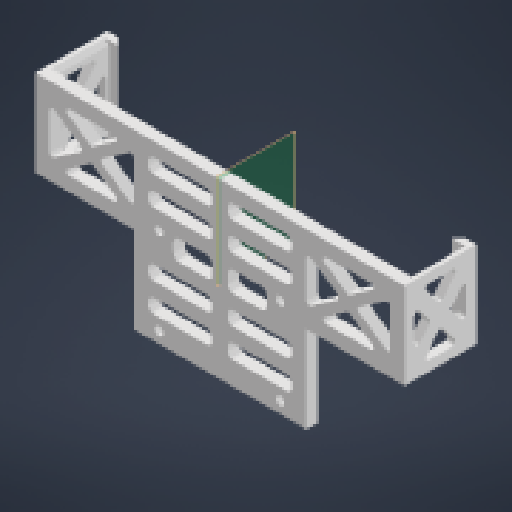
# Autodesk Inventor part: Mux_switch_holder
Saved by Autodesk Inventor 2026.1 (Build 301233020, 233B)
## iProperties
Created: 2025-10-27
Part Number: Mux_switch_holder
Material: Generic
Document SubType Name: Modeling
Designer: Mikke
Density: 1 g/cm^3
Appearance: Default
Author: Mikke
Autodesk Inventor part; units mm, degrees
(part 1 of 2)
ref_plane "YZ Plane" through (0, 0, 0) normal (1, 0, 0) x (0, 1, 0)
ref_plane "XZ Plane" through (0, 0, 0) normal (0, 1, 0) x (-1, 0, 0)
ref_plane "XY Plane" through (0, 0, 0) normal (0, 0, 1) x (1, 0, 0)
sketch "Sketch1" plane through (0, 0, 0) normal (0, 0, 1) x (1, 0, 0)
  line L0 (44.8879, -29.1603) -> (44.2305, -29.1603) projected
  line L1 (44.2305, -29.1603) -> (44.2305, -28.4336) projected
  line L2 (44.2305, -28.4336) -> (42.1345, -28.4336) projected
  line L3 (42.1345, -28.4336) -> (42.1345, -27.6476) projected
  line L4 (42.1345, -27.6476) -> (44.2305, -27.6476) projected
  line L5 (44.2305, -27.6476) -> (44.2305, -24.9536) projected
  line L6 (44.2305, -24.9536) -> (45.0906, -24.9536) projected
  line L7 (45.0906, -24.9536) -> (48.2345, -27.6822) projected
  line L8 (48.2345, -27.6822) -> (48.2345, -28.4336) projected
  line L9 (48.2345, -28.4336) -> (44.8879, -28.4336) projected
  line L10 (44.8879, -28.4336) -> (44.8879, -29.1603) projected
  line L11 (44.4529, -11.8242) -> (42.1345, -13.4011) projected
  line L12 (42.1345, -13.4011) -> (42.1345, -12.457) projected
  line L13 (42.1345, -12.457) -> (43.8548, -11.3447) projected
  line L14 (43.8548, -11.3447) -> (42.1345, -10.2028) projected
  line L15 (42.1345, -10.2028) -> (42.1345, -9.3279) projected
  line L16 (42.1345, -9.3279) -> (44.4035, -10.9147) projected
  line L17 (44.4035, -10.9147) -> (46.712, -9.3427) projected
  line L18 (46.712, -9.3427) -> (46.712, -10.2869) projected
  line L19 (46.712, -10.2869) -> (45.0065, -11.3942) projected
  line L20 (45.0065, -11.3942) -> (46.712, -12.5262) projected
  line L21 (46.712, -12.5262) -> (46.712, -13.4011) projected
  line L22 (46.712, -13.4011) -> (44.4529, -11.8242) projected
  line L23 (46.712, -8.7149) -> (42.1345, -8.7149) projected
  line L24 (42.1345, -8.7149) -> (42.1345, -7.9438) projected
  line L25 (42.1345, -7.9438) -> (46.712, -7.9438) projected
  line L26 (46.712, -7.9438) -> (46.712, -8.7149) projected
  spline S0 degree 2 poles (42.1741, -4.3352) (42.1147, -4.1177) (42.0455, -3.6728) (42.0455, -3.48) knots 0 0 0 1 2 2 2 projected
  spline S1 degree 2 poles (42.0455, -3.48) (42.0455, -2.8522) (42.7623, -2.1453) (43.5384, -2.1453) knots 0 0 0 1 2 2 2 projected
  line L27 (43.5384, -2.1453) -> (46.0743, -2.1453) projected
  line L28 (46.0743, -2.1453) -> (46.0743, -1.6262) projected
  line L29 (46.0743, -1.6262) -> (46.712, -1.6262) projected
  line L30 (46.712, -1.6262) -> (46.712, -2.1453) projected
  line L31 (46.712, -2.1453) -> (48.0269, -2.1453) projected
  line L32 (48.0269, -2.1453) -> (48.0269, -2.9164) projected
  line L33 (48.0269, -2.9164) -> (46.712, -2.9164) projected
  line L34 (46.712, -2.9164) -> (46.712, -4.3352) projected
  line L35 (46.712, -4.3352) -> (46.0743, -4.3352) projected
  line L36 (46.0743, -4.3352) -> (46.0743, -2.9164) projected
  line L37 (46.0743, -2.9164) -> (43.8943, -2.9164) projected
  spline S2 degree 2 poles (43.8943, -2.9164) (43.5483, -2.9164) (43.1676, -2.9412) (43.0045, -3.0252) knots 0 0 0 1 2 2 2 projected
  spline S3 degree 2 poles (43.0045, -3.0252) (42.8612, -3.0944) (42.7178, -3.4058) (42.7178, -3.6728) knots 0 0 0 1 2 2 2 projected
  spline S4 degree 2 poles (42.7178, -3.6728) (42.7178, -3.8606) (42.8315, -4.2116) (42.8661, -4.2907) knots 0 0 0 1 2 2 2 projected
  line L38 (42.8661, -4.2907) -> (42.8661, -4.3352) projected
  line L39 (42.8661, -4.3352) -> (42.1741, -4.3352) projected
  line L40 (42.1345, -0.2421) -> (42.6189, -0.2421) projected
  spline S5 degree 2 poles (42.6189, -0.2421) (42.5497, -0.1482) (42.3026, 0.1682) (42.2284, 0.3165) knots 0 0 0 1 2 2 2 projected
  spline S6 degree 2 poles (42.2284, 0.3165) (42.1197, 0.5191) (42.006, 0.8998) (42.006, 1.2458) knots 0 0 0 1 2 2 2 projected
  spline S7 degree 2 poles (42.006, 1.2458) (42.006, 1.5276) (42.2185, 2.0367) (42.4113, 2.2295) knots 0 0 0 1 2 2 2 projected
  spline S8 degree 2 poles (42.4113, 2.2295) (42.5992, 2.4124) (43.1528, 2.6349) (43.4593, 2.6349) knots 0 0 0 1 2 2 2 projected
  spline S9 degree 2 poles (43.4593, 2.6349) (43.9339, 2.6349) (44.6061, 2.2344) (44.7989, 1.7994) knots 0 0 0 1 2 2 2 projected
  spline S10 degree 2 poles (44.7989, 1.7994) (44.9769, 1.4139) (45.1104, 0.3659) (45.145, -0.2421) knots 0 0 0 1 2 2 2 projected
  line L41 (45.145, -0.2421) -> (45.2933, -0.2421) projected
  spline S11 degree 2 poles (45.2933, -0.2421) (45.5602, -0.2421) (45.8914, -0.079) (45.9853, 0.0693) knots 0 0 0 1 2 2 2 projected
  spline S12 degree 2 poles (45.9853, 0.0693) (46.0792, 0.2176) (46.1386, 0.6427) (46.1386, 0.8701) knots 0 0 0 1 2 2 2 projected
  spline S13 degree 2 poles (46.1386, 0.8701) (46.1386, 1.137) (45.9804, 1.8588) (45.8271, 2.2196) knots 0 0 0 1 2 2 2 projected
  line L42 (45.8271, 2.2196) -> (45.8271, 2.2641) projected
  line L43 (45.8271, 2.2641) -> (46.6131, 2.2641) projected
  spline S14 degree 2 poles (46.6131, 2.2641) (46.6724, 2.0515) (46.8207, 1.2557) (46.8207, 0.8652) knots 0 0 0 1 2 2 2 projected
  spline S15 degree 2 poles (46.8207, 0.8652) (46.8207, 0.3906) (46.6724, -0.257) (46.4796, -0.514) knots 0 0 0 1 2 2 2 projected
  spline S16 degree 2 poles (46.4796, -0.514) (46.2918, -0.7661) (45.6937, -1.0133) (45.2636, -1.0133) knots 0 0 0 1 2 2 2 projected
  line L44 (45.2636, -1.0133) -> (42.1345, -1.0133) projected
  line L45 (42.1345, -1.0133) -> (42.1345, -0.2421) projected
  line L46 (46.6873, 11.9925) -> (45.8865, 11.9925) projected
  line L47 (45.8865, 11.9925) -> (45.8865, 12.032) projected
  spline S17 degree 2 poles (45.8865, 12.032) (45.9112, 12.121) (45.9211, 12.3138) (45.9211, 12.4473) knots 0 0 0 1 2 2 2 projected
  spline S18 degree 2 poles (45.9211, 12.4473) (45.9211, 12.7587) (45.6492, 13.3716) (45.3822, 13.6485) knots 0 0 0 1 2 2 2 projected
  line L48 (45.3822, 13.6485) -> (42.1345, 13.6485) projected
  line L49 (42.1345, 13.6485) -> (42.1345, 14.4196) projected
  line L50 (42.1345, 14.4196) -> (46.712, 14.4196) projected
  line L51 (46.712, 14.4196) -> (46.712, 13.6485) projected
  line L52 (46.712, 13.6485) -> (46.0298, 13.6485) projected
  spline S19 degree 2 poles (46.0298, 13.6485) (46.4055, 13.2283) (46.712, 12.6005) (46.712, 12.3039) knots 0 0 0 1 2 2 2 projected
  spline S20 degree 2 poles (46.712, 12.3039) (46.712, 12.1853) (46.7021, 12.0666) (46.6873, 11.9925) knots 0 0 0 1 2 2 2 projected
  spline S21 degree 2 poles (42.1592, 15.9817) (42.095, 16.2041) (42.0307, 16.5699) (42.0307, 16.8468) knots 0 0 0 1 2 2 2 projected
  spline S22 degree 2 poles (42.0307, 16.8468) (42.0307, 17.9442) (43.2616, 19.1503) (44.3985, 19.1503) knots 0 0 0 1 2 2 2 projected
  spline S23 degree 2 poles (44.3985, 19.1503) (45.5157, 19.1503) (46.8405, 17.9788) (46.8405, 17.0346) knots 0 0 0 1 2 2 2 projected
  spline S24 degree 2 poles (46.8405, 17.0346) (46.8405, 16.6095) (46.5933, 15.952) (46.3313, 15.7098) knots 0 0 0 1 2 2 2 projected
  spline S25 degree 2 poles (46.3313, 15.7098) (46.0694, 15.4626) (45.313, 15.2007) (44.7643, 15.2007) knots 0 0 0 1 2 2 2 projected
  line L53 (44.7643, 15.2007) -> (44.3441, 15.2007) projected
  line L54 (44.3441, 15.2007) -> (44.3441, 18.3693) projected
  spline S26 degree 2 poles (44.3441, 18.3693) (43.5483, 18.3693) (42.703, 17.5685) (42.703, 16.8567) knots 0 0 0 1 2 2 2 projected
  spline S27 degree 2 poles (42.703, 16.8567) (42.703, 16.6045) (42.8167, 16.1152) (42.9057, 15.9174) knots 0 0 0 1 2 2 2 projected
  spline S28 degree 2 poles (42.9057, 15.9174) (43.0045, 15.7098) (43.1775, 15.4231) (43.2566, 15.3292) knots 0 0 0 1 2 2 2 projected
  line L55 (43.2566, 15.3292) -> (43.2566, 15.2847) projected
  line L56 (43.2566, 15.2847) -> (42.4163, 15.2847) projected
  spline S29 degree 2 poles (42.4163, 15.2847) (42.3619, 15.4182) (42.2037, 15.8235) (42.1592, 15.9817) knots 0 0 0 1 2 2 2 projected
  spline S30 degree 2 poles (42.1741, 21.3204) (42.1147, 21.5379) (42.0455, 21.9828) (42.0455, 22.1756) knots 0 0 0 1 2 2 2 projected
  spline S31 degree 2 poles (42.0455, 22.1756) (42.0455, 22.8034) (42.7623, 23.5103) (43.5384, 23.5103) knots 0 0 0 1 2 2 2 projected
  line L57 (43.5384, 23.5103) -> (46.0743, 23.5103) projected
  line L58 (46.0743, 23.5103) -> (46.0743, 24.0293) projected
  line L59 (46.0743, 24.0293) -> (46.712, 24.0293) projected
  line L60 (46.712, 24.0293) -> (46.712, 23.5103) projected
  line L61 (46.712, 23.5103) -> (48.0269, 23.5103) projected
  line L62 (48.0269, 23.5103) -> (48.0269, 22.7391) projected
  line L63 (48.0269, 22.7391) -> (46.712, 22.7391) projected
  line L64 (46.712, 22.7391) -> (46.712, 21.3204) projected
  line L65 (46.712, 21.3204) -> (46.0743, 21.3204) projected
  line L66 (46.0743, 21.3204) -> (46.0743, 22.7391) projected
  line L67 (46.0743, 22.7391) -> (43.8943, 22.7391) projected
  spline S32 degree 2 poles (43.8943, 22.7391) (43.5483, 22.7391) (43.1676, 22.7144) (43.0045, 22.6304) knots 0 0 0 1 2 2 2 projected
  spline S33 degree 2 poles (43.0045, 22.6304) (42.8612, 22.5612) (42.7178, 22.2498) (42.7178, 21.9828) knots 0 0 0 1 2 2 2 projected
  spline S34 degree 2 poles (42.7178, 21.9828) (42.7178, 21.795) (42.8315, 21.444) (42.8661, 21.3649) knots 0 0 0 1 2 2 2 projected
  line L68 (42.8661, 21.3649) -> (42.8661, 21.3204) projected
  line L69 (42.8661, 21.3204) -> (42.1741, 21.3204) projected
  spline S35 degree 2 poles (45.5256, 30.1244) (45.3773, 29.5806) (44.5913, 28.9825) (44.008, 28.9825) knots 0 0 0 1 2 2 2 projected
  spline S36 degree 2 poles (44.008, 28.9825) (43.5532, 28.9825) (42.8562, 29.3285) (42.6288, 29.6152) knots 0 0 0 1 2 2 2 projected
  spline S37 degree 2 poles (42.6288, 29.6152) (42.3619, 29.9613) (42.1345, 30.7473) (42.1345, 31.3701) knots 0 0 0 1 2 2 2 projected
  line L70 (42.1345, 31.3701) -> (42.1345, 33.12) projected
  line L71 (42.1345, 33.12) -> (48.2345, 33.12) projected
  line L72 (48.2345, 33.12) -> (48.2345, 31.5036) projected
  spline S38 degree 2 poles (48.2345, 31.5036) (48.2345, 30.8511) (48.1505, 30.1985) (47.9873, 29.902) knots 0 0 0 1 2 2 2 projected
  spline S39 degree 2 poles (47.9873, 29.902) (47.8143, 29.5708) (47.2459, 29.2692) (46.8603, 29.2692) knots 0 0 0 1 2 2 2 projected
  spline S40 degree 2 poles (46.8603, 29.2692) (46.4302, 29.2692) (45.748, 29.724) (45.5553, 30.1244) knots 0 0 0 1 2 2 2 projected
  line L73 (45.5553, 30.1244) -> (45.5256, 30.1244) projected
  line L74 (52.8849, -32.3388) -> (52.178, -32.3388) projected
  line L75 (52.178, -32.3388) -> (52.178, -28.577) projected
  line L76 (52.178, -28.577) -> (53.0431, -28.577) projected
  spline S41 degree 2 poles (53.0431, -28.577) (53.4237, -28.9823) (54.1306, -29.704) (54.5112, -30.0501) knots 0 0 0 1 2 2 2 projected
  spline S42 degree 2 poles (54.5112, -30.0501) (55.2774, -30.7471) (56.1969, -31.2562) (56.6863, -31.2562) knots 0 0 0 1 2 2 2 projected
  spline S43 degree 2 poles (56.6863, -31.2562) (56.9433, -31.2562) (57.3289, -31.098) (57.4525, -30.9547) knots 0 0 0 1 2 2 2 projected
  spline S44 degree 2 poles (57.4525, -30.9547) (57.5761, -30.8113) (57.6996, -30.4357) (57.6996, -30.2083) knots 0 0 0 1 2 2 2 projected
  spline S45 degree 2 poles (57.6996, -30.2083) (57.6996, -29.9908) (57.5909, -29.5459) (57.5068, -29.3432) knots 0 0 0 1 2 2 2 projected
  spline S46 degree 2 poles (57.5068, -29.3432) (57.4376, -29.1702) (57.2399, -28.8489) (57.1707, -28.75) knots 0 0 0 1 2 2 2 projected
  line L77 (57.1707, -28.75) -> (57.1707, -28.7055) projected
  line L78 (57.1707, -28.7055) -> (58.0407, -28.7055) projected
  spline S47 degree 2 poles (58.0407, -28.7055) (58.1643, -28.9576) (58.4065, -29.8622) (58.4065, -30.2676) knots 0 0 0 1 2 2 2 projected
  spline S48 degree 2 poles (58.4065, -30.2676) (58.4065, -31.1228) (57.5019, -32.0867) (56.7308, -32.0867) knots 0 0 0 1 2 2 2 projected
  spline S49 degree 2 poles (56.7308, -32.0867) (56.3699, -32.0867) (55.7668, -31.9186) (55.5098, -31.7703) knots 0 0 0 1 2 2 2 projected
  spline S50 degree 2 poles (55.5098, -31.7703) (55.2428, -31.622) (54.7188, -31.192) (54.4667, -30.9547) knots 0 0 0 1 2 2 2 projected
  spline S51 degree 2 poles (54.4667, -30.9547) (54.0466, -30.5691) (53.1469, -29.625) (52.8849, -29.3432) knots 0 0 0 1 2 2 2 projected
  line L79 (52.8849, -29.3432) -> (52.8849, -32.3388) projected
  line L80 (55.2181, -23.1888) -> (54.4766, -23.1888) projected
  line L81 (54.4766, -23.1888) -> (54.4766, -20.8803) projected
  line L82 (54.4766, -20.8803) -> (55.2181, -20.8803) projected
  line L83 (55.2181, -20.8803) -> (55.2181, -23.1888) projected
  line L84 (55.2181, -15.5663) -> (54.4766, -15.5663) projected
  line L85 (54.4766, -15.5663) -> (54.4766, -13.2578) projected
  line L86 (54.4766, -13.2578) -> (55.2181, -13.2578) projected
  line L87 (55.2181, -13.2578) -> (55.2181, -15.5663) projected
  line L88 (52.178, -7.9438) -> (52.178, -4.1275) projected
  line L89 (52.178, -4.1275) -> (58.278, -4.1275) projected
  line L90 (58.278, -4.1275) -> (58.278, -7.9438) projected
  line L91 (58.278, -7.9438) -> (57.5563, -7.9438) projected
  line L92 (57.5563, -7.9438) -> (57.5563, -4.9382) projected
  line L93 (57.5563, -4.9382) -> (55.8855, -4.9382) projected
  line L94 (55.8855, -4.9382) -> (55.8855, -7.7411) projected
  line L95 (55.8855, -7.7411) -> (55.1637, -7.7411) projected
  line L96 (55.1637, -7.7411) -> (55.1637, -4.9382) projected
  line L97 (55.1637, -4.9382) -> (52.8997, -4.9382) projected
  line L98 (52.8997, -4.9382) -> (52.8997, -7.9438) projected
  line L99 (52.8997, -7.9438) -> (52.178, -7.9438) projected
  line L100 (52.8008, 10.1931) -> (52.178, 10.1931) projected
  line L101 (52.178, 10.1931) -> (52.178, 13.169) projected
  line L102 (52.178, 13.169) -> (52.8008, 13.169) projected
  line L103 (52.8008, 13.169) -> (52.8008, 12.0617) projected
  line L104 (52.8008, 12.0617) -> (56.8889, 12.0617) projected
  line L105 (56.8889, 12.0617) -> (56.8889, 13.169) projected
  line L106 (56.8889, 13.169) -> (57.4475, 13.169) projected
  spline S52 degree 2 poles (57.4475, 13.169) (57.4475, 12.5412) (57.8034, 11.948) (58.2978, 11.9084) knots 0 0 0 1 2 2 2 projected
  line L107 (58.2978, 11.9084) -> (58.2978, 11.2757) projected
  line L108 (58.2978, 11.2757) -> (52.8008, 11.2757) projected
  line L109 (52.8008, 11.2757) -> (52.8008, 10.1931) projected
  spline S53 degree 2 poles (52.6229, 25.1218) (52.356, 25.4135) (52.0692, 26.155) (52.0692, 26.7135) knots 0 0 0 1 2 2 2 projected
  spline S54 degree 2 poles (52.0692, 26.7135) (52.0692, 27.3759) (52.3461, 28.3053) (52.5438, 28.7156) knots 0 0 0 1 2 2 2 projected
  line L110 (52.5438, 28.7156) -> (53.5621, 28.7156) projected
  line L111 (53.5621, 28.7156) -> (53.5621, 28.6562) projected
  spline S55 degree 2 poles (53.5621, 28.6562) (53.1864, 28.2558) (52.7712, 27.2425) (52.7712, 26.7729) knots 0 0 0 1 2 2 2 projected
  spline S56 degree 2 poles (52.7712, 26.7729) (52.7712, 26.1006) (53.3298, 25.4135) (53.7895, 25.4135) knots 0 0 0 1 2 2 2 projected
  spline S57 degree 2 poles (53.7895, 25.4135) (54.1553, 25.4135) (54.6101, 25.7743) (54.7238, 26.1648) knots 0 0 0 1 2 2 2 projected
  spline S58 degree 2 poles (54.7238, 26.1648) (54.8029, 26.4466) (54.9116, 26.9162) (55.0006, 27.2672) knots 0 0 0 1 2 2 2 projected
  spline S59 degree 2 poles (55.0006, 27.2672) (55.0846, 27.5836) (55.3367, 28.0828) (55.5394, 28.2756) knots 0 0 0 1 2 2 2 projected
  spline S60 degree 2 poles (55.5394, 28.2756) (55.7421, 28.4635) (56.2859, 28.6711) (56.6418, 28.6711) knots 0 0 0 1 2 2 2 projected
  spline S61 degree 2 poles (56.6418, 28.6711) (57.3833, 28.6711) (58.3867, 27.5144) (58.3867, 26.6196) knots 0 0 0 1 2 2 2 projected
  spline S62 degree 2 poles (58.3867, 26.6196) (58.3867, 26.1055) (58.1841, 25.196) (57.9913, 24.8054) knots 0 0 0 1 2 2 2 projected
  line L112 (57.9913, 24.8054) -> (57.0224, 24.8054) projected
  line L113 (57.0224, 24.8054) -> (57.0224, 24.8648) projected
  spline S63 degree 2 poles (57.0224, 24.8648) (57.2893, 25.1564) (57.6848, 26.066) (57.6848, 26.5652) knots 0 0 0 1 2 2 2 projected
  spline S64 degree 2 poles (57.6848, 26.5652) (57.6848, 27.1288) (57.1559, 27.8258) (56.7258, 27.8258) knots 0 0 0 1 2 2 2 projected
  spline S65 degree 2 poles (56.7258, 27.8258) (56.3402, 27.8258) (55.8805, 27.4155) (55.7767, 27.0299) knots 0 0 0 1 2 2 2 projected
  spline S66 degree 2 poles (55.7767, 27.0299) (55.7075, 26.7729) (55.5295, 26.0264) (55.4554, 25.7793) knots 0 0 0 1 2 2 2 projected
  spline S67 degree 2 poles (55.4554, 25.7793) (55.2626, 25.1515) (54.4865, 24.5682) (53.918, 24.5682) knots 0 0 0 1 2 2 2 projected
  spline S68 degree 2 poles (53.918, 24.5682) (53.5572, 24.5682) (52.8651, 24.8598) (52.6229, 25.1218) knots 0 0 0 1 2 2 2 projected
  line L114 (52.178, 29.3038) -> (52.178, 33.12) projected
  line L115 (52.178, 33.12) -> (58.278, 33.12) projected
  line L116 (58.278, 33.12) -> (58.278, 29.3038) projected
  line L117 (58.278, 29.3038) -> (57.5563, 29.3038) projected
  line L118 (57.5563, 29.3038) -> (57.5563, 32.3093) projected
  line L119 (57.5563, 32.3093) -> (55.8855, 32.3093) projected
  line L120 (55.8855, 32.3093) -> (55.8855, 29.5065) projected
  line L121 (55.8855, 29.5065) -> (55.1637, 29.5065) projected
  line L122 (55.1637, 29.5065) -> (55.1637, 32.3093) projected
  line L123 (55.1637, 32.3093) -> (52.8997, 32.3093) projected
  line L124 (52.8997, 32.3093) -> (52.8997, 29.3038) projected
  line L125 (52.8997, 29.3038) -> (52.178, 29.3038) projected
  spline S69 degree 2 poles (57.7936, 20.1686) (57.403, 19.5804) (56.1128, 18.9328) (55.2231, 18.9328) knots 0 0 0 1 2 2 2 projected
  spline S70 degree 2 poles (55.2231, 18.9328) (54.3876, 18.9328) (53.0431, 19.6101) (52.6674, 20.1785) knots 0 0 0 1 2 2 2 projected
  spline S71 degree 2 poles (52.6674, 20.1785) (52.3757, 20.6432) (52.178, 21.5973) (52.178, 22.3387) knots 0 0 0 1 2 2 2 projected
  line L126 (52.178, 22.3387) -> (52.178, 23.7426) projected
  line L127 (52.178, 23.7426) -> (58.278, 23.7426) projected
  line L128 (58.278, 23.7426) -> (58.278, 22.3536) projected
  spline S72 degree 2 poles (58.278, 22.3536) (58.278, 21.4934) (58.0209, 20.5147) (57.7936, 20.1686) knots 0 0 0 1 2 2 2 projected
  spline S73 degree 2 poles (55.5889, 15.1562) (55.3615, 14.8546) (54.6694, 14.5284) (54.1158, 14.5284) knots 0 0 0 1 2 2 2 projected
  spline S74 degree 2 poles (54.1158, 14.5284) (53.6758, 14.5284) (52.9244, 14.8101) (52.6476, 15.0672) knots 0 0 0 1 2 2 2 projected
  spline S75 degree 2 poles (52.6476, 15.0672) (52.3708, 15.3242) (52.0495, 16.0904) (52.0495, 16.565) knots 0 0 0 1 2 2 2 projected
  spline S76 degree 2 poles (52.0495, 16.565) (52.0495, 17) (52.2423, 17.8503) (52.3955, 18.1617) knots 0 0 0 1 2 2 2 projected
  line L129 (52.3955, 18.1617) -> (53.2606, 18.1617) projected
  line L130 (53.2606, 18.1617) -> (53.2606, 18.1024) projected
  spline S77 degree 2 poles (53.2606, 18.1024) (53.1914, 18.0084) (53.0134, 17.6575) (52.9343, 17.4449) knots 0 0 0 1 2 2 2 projected
  spline S78 degree 2 poles (52.9343, 17.4449) (52.8503, 17.2027) (52.7564, 16.8023) (52.7564, 16.5502) knots 0 0 0 1 2 2 2 projected
  spline S79 degree 2 poles (52.7564, 16.5502) (52.7564, 16.303) (52.9343, 15.8383) (53.1271, 15.6703) knots 0 0 0 1 2 2 2 projected
  spline S80 degree 2 poles (53.1271, 15.6703) (53.31, 15.517) (53.7944, 15.3588) (54.1207, 15.3588) knots 0 0 0 1 2 2 2 projected
  spline S81 degree 2 poles (54.1207, 15.3588) (54.447, 15.3588) (54.8622, 15.5368) (55.0006, 15.7049) knots 0 0 0 1 2 2 2 projected
  spline S82 degree 2 poles (55.0006, 15.7049) (55.1538, 15.8779) (55.2824, 16.392) (55.2824, 16.7034) knots 0 0 0 1 2 2 2 projected
  spline S83 degree 2 poles (55.2824, 16.7034) (55.2824, 17.0396) (55.1786, 17.7069) (55.1341, 17.9096) knots 0 0 0 1 2 2 2 projected
  line L131 (55.1341, 17.9096) -> (58.278, 17.9096) projected
  line L132 (58.278, 17.9096) -> (58.278, 14.563) projected
  line L133 (58.278, 14.563) -> (57.5612, 14.563) projected
  line L134 (57.5612, 14.563) -> (57.5612, 17.1236) projected
  line L135 (57.5612, 17.1236) -> (55.9349, 17.1236) projected
  spline S84 degree 2 poles (55.9349, 17.1236) (55.9547, 16.9753) (55.9695, 16.6886) (55.9695, 16.5699) knots 0 0 0 1 2 2 2 projected
  spline S85 degree 2 poles (55.9695, 16.5699) (55.9695, 16.1003) (55.8162, 15.4528) (55.5889, 15.1562) knots 0 0 0 1 2 2 2 projected
  spline S86 degree 2 poles (58.4016, 7.2222) (58.4016, 6.2187) (56.8197, 5.2746) (55.228, 5.2746) knots 0 0 0 1 2 2 2 projected
  spline S87 degree 2 poles (55.228, 5.2746) (53.5868, 5.2746) (52.0495, 6.2286) (52.0495, 7.2222) knots 0 0 0 1 2 2 2 projected
  spline S88 degree 2 poles (52.0495, 7.2222) (52.0495, 8.2306) (53.6165, 9.1748) (55.2231, 9.1748) knots 0 0 0 1 2 2 2 projected
  spline S89 degree 2 poles (55.2231, 9.1748) (56.8741, 9.1748) (58.4016, 8.2208) (58.4016, 7.2222) knots 0 0 0 1 2 2 2 projected
  line L136 (58.5499, 0.0396) -> (58.5499, -0.6623) projected
  line L137 (58.5499, -0.6623) -> (50.8532, 1.7253) projected
  line L138 (50.8532, 1.7253) -> (50.8532, 2.4173) projected
  line L139 (50.8532, 2.4173) -> (58.5499, 0.0396) projected
  spline S90 degree 2 poles (52.6229, -12.1258) (52.356, -11.8341) (52.0692, -11.0926) (52.0692, -10.534) knots 0 0 0 1 2 2 2 projected
  spline S91 degree 2 poles (52.0692, -10.534) (52.0692, -9.8716) (52.3461, -8.9423) (52.5438, -8.532) knots 0 0 0 1 2 2 2 projected
  line L140 (52.5438, -8.532) -> (53.5621, -8.532) projected
  line L141 (53.5621, -8.532) -> (53.5621, -8.5913) projected
  spline S92 degree 2 poles (53.5621, -8.5913) (53.1864, -8.9917) (52.7712, -10.0051) (52.7712, -10.4747) knots 0 0 0 1 2 2 2 projected
  spline S93 degree 2 poles (52.7712, -10.4747) (52.7712, -11.147) (53.3298, -11.8341) (53.7895, -11.8341) knots 0 0 0 1 2 2 2 projected
  spline S94 degree 2 poles (53.7895, -11.8341) (54.1553, -11.8341) (54.6101, -11.4733) (54.7238, -11.0827) knots 0 0 0 1 2 2 2 projected
  spline S95 degree 2 poles (54.7238, -11.0827) (54.8029, -10.801) (54.9116, -10.3314) (55.0006, -9.9804) knots 0 0 0 1 2 2 2 projected
  spline S96 degree 2 poles (55.0006, -9.9804) (55.0846, -9.664) (55.3367, -9.1647) (55.5394, -8.972) knots 0 0 0 1 2 2 2 projected
  spline S97 degree 2 poles (55.5394, -8.972) (55.7421, -8.7841) (56.2859, -8.5765) (56.6418, -8.5765) knots 0 0 0 1 2 2 2 projected
  spline S98 degree 2 poles (56.6418, -8.5765) (57.3833, -8.5765) (58.3867, -9.7332) (58.3867, -10.628) knots 0 0 0 1 2 2 2 projected
  spline S99 degree 2 poles (58.3867, -10.628) (58.3867, -11.1421) (58.1841, -12.0516) (57.9913, -12.4421) knots 0 0 0 1 2 2 2 projected
  line L142 (57.9913, -12.4421) -> (57.0224, -12.4421) projected
  line L143 (57.0224, -12.4421) -> (57.0224, -12.3828) projected
  spline S100 degree 2 poles (57.0224, -12.3828) (57.2893, -12.0912) (57.6848, -11.1816) (57.6848, -10.6823) knots 0 0 0 1 2 2 2 projected
  spline S101 degree 2 poles (57.6848, -10.6823) (57.6848, -10.1188) (57.1559, -9.4218) (56.7258, -9.4218) knots 0 0 0 1 2 2 2 projected
  spline S102 degree 2 poles (56.7258, -9.4218) (56.3402, -9.4218) (55.8805, -9.8321) (55.7767, -10.2177) knots 0 0 0 1 2 2 2 projected
  spline S103 degree 2 poles (55.7767, -10.2177) (55.7075, -10.4747) (55.5295, -11.2211) (55.4554, -11.4683) knots 0 0 0 1 2 2 2 projected
  spline S104 degree 2 poles (55.4554, -11.4683) (55.2626, -12.0961) (54.4865, -12.6794) (53.918, -12.6794) knots 0 0 0 1 2 2 2 projected
  spline S105 degree 2 poles (53.918, -12.6794) (53.5572, -12.6794) (52.8651, -12.3878) (52.6229, -12.1258) knots 0 0 0 1 2 2 2 projected
  spline S106 degree 2 poles (55.5889, -19.4468) (55.3615, -19.7483) (54.6694, -20.0745) (54.1158, -20.0745) knots 0 0 0 1 2 2 2 projected
  spline S107 degree 2 poles (54.1158, -20.0745) (53.6758, -20.0745) (52.9244, -19.7928) (52.6476, -19.5357) knots 0 0 0 1 2 2 2 projected
  spline S108 degree 2 poles (52.6476, -19.5357) (52.3708, -19.2787) (52.0495, -18.5125) (52.0495, -18.0379) knots 0 0 0 1 2 2 2 projected
  spline S109 degree 2 poles (52.0495, -18.0379) (52.0495, -17.6029) (52.2423, -16.7527) (52.3955, -16.4412) knots 0 0 0 1 2 2 2 projected
  line L144 (52.3955, -16.4412) -> (53.2606, -16.4412) projected
  line L145 (53.2606, -16.4412) -> (53.2606, -16.5006) projected
  spline S110 degree 2 poles (53.2606, -16.5006) (53.1914, -16.5945) (53.0134, -16.9455) (52.9343, -17.158) knots 0 0 0 1 2 2 2 projected
  spline S111 degree 2 poles (52.9343, -17.158) (52.8503, -17.4002) (52.7564, -17.8006) (52.7564, -18.0527) knots 0 0 0 1 2 2 2 projected
  spline S112 degree 2 poles (52.7564, -18.0527) (52.7564, -18.2999) (52.9343, -18.7646) (53.1271, -18.9327) knots 0 0 0 1 2 2 2 projected
  spline S113 degree 2 poles (53.1271, -18.9327) (53.31, -19.0859) (53.7944, -19.2441) (54.1207, -19.2441) knots 0 0 0 1 2 2 2 projected
  spline S114 degree 2 poles (54.1207, -19.2441) (54.447, -19.2441) (54.8622, -19.0661) (55.0006, -18.898) knots 0 0 0 1 2 2 2 projected
  spline S115 degree 2 poles (55.0006, -18.898) (55.1538, -18.725) (55.2824, -18.2109) (55.2824, -17.8995) knots 0 0 0 1 2 2 2 projected
  spline S116 degree 2 poles (55.2824, -17.8995) (55.2824, -17.5634) (55.1786, -16.896) (55.1341, -16.6933) knots 0 0 0 1 2 2 2 projected
  line L146 (55.1341, -16.6933) -> (58.278, -16.6933) projected
  line L147 (58.278, -16.6933) -> (58.278, -20.0399) projected
  line L148 (58.278, -20.0399) -> (57.5612, -20.0399) projected
  line L149 (57.5612, -20.0399) -> (57.5612, -17.4793) projected
  line L150 (57.5612, -17.4793) -> (55.9349, -17.4793) projected
  spline S117 degree 2 poles (55.9349, -17.4793) (55.9547, -17.6276) (55.9695, -17.9143) (55.9695, -18.033) knots 0 0 0 1 2 2 2 projected
  spline S118 degree 2 poles (55.9695, -18.033) (55.9695, -18.5026) (55.8162, -19.1502) (55.5889, -19.4468) knots 0 0 0 1 2 2 2 projected
  line L151 (52.8008, -27.4549) -> (52.178, -27.4549) projected
  line L152 (52.178, -27.4549) -> (52.178, -24.479) projected
  line L153 (52.178, -24.479) -> (52.8008, -24.479) projected
  line L154 (52.8008, -24.479) -> (52.8008, -25.5863) projected
  line L155 (52.8008, -25.5863) -> (56.8889, -25.5863) projected
  line L156 (56.8889, -25.5863) -> (56.8889, -24.479) projected
  line L157 (56.8889, -24.479) -> (57.4475, -24.479) projected
  spline S119 degree 2 poles (57.4475, -24.479) (57.4475, -25.1068) (57.8034, -25.7) (58.2978, -25.7395) knots 0 0 0 1 2 2 2 projected
  line L158 (58.2978, -25.7395) -> (58.2978, -26.3723) projected
  line L159 (58.2978, -26.3723) -> (52.8008, -26.3723) projected
  line L160 (52.8008, -26.3723) -> (52.8008, -27.4549) projected
  line L161 (52.8849, -36.9163) -> (52.178, -36.9163) projected
  line L162 (52.178, -36.9163) -> (52.178, -33.1545) projected
  line L163 (52.178, -33.1545) -> (53.0431, -33.1545) projected
  spline S120 degree 2 poles (53.0431, -33.1545) (53.4237, -33.5598) (54.1306, -34.2815) (54.5112, -34.6275) knots 0 0 0 1 2 2 2 projected
  spline S121 degree 2 poles (54.5112, -34.6275) (55.2774, -35.3245) (56.1969, -35.8337) (56.6863, -35.8337) knots 0 0 0 1 2 2 2 projected
  spline S122 degree 2 poles (56.6863, -35.8337) (56.9433, -35.8337) (57.3289, -35.6755) (57.4525, -35.5322) knots 0 0 0 1 2 2 2 projected
  spline S123 degree 2 poles (57.4525, -35.5322) (57.5761, -35.3888) (57.6996, -35.0131) (57.6996, -34.7857) knots 0 0 0 1 2 2 2 projected
  spline S124 degree 2 poles (57.6996, -34.7857) (57.6996, -34.5682) (57.5909, -34.1233) (57.5068, -33.9207) knots 0 0 0 1 2 2 2 projected
  spline S125 degree 2 poles (57.5068, -33.9207) (57.4376, -33.7476) (57.2399, -33.4263) (57.1707, -33.3275) knots 0 0 0 1 2 2 2 projected
  line L164 (57.1707, -33.3275) -> (57.1707, -33.283) projected
  line L165 (57.1707, -33.283) -> (58.0407, -33.283) projected
  spline S126 degree 2 poles (58.0407, -33.283) (58.1643, -33.5351) (58.4065, -34.4397) (58.4065, -34.8451) knots 0 0 0 1 2 2 2 projected
  spline S127 degree 2 poles (58.4065, -34.8451) (58.4065, -35.7002) (57.5019, -36.6642) (56.7308, -36.6642) knots 0 0 0 1 2 2 2 projected
  spline S128 degree 2 poles (56.7308, -36.6642) (56.3699, -36.6642) (55.7668, -36.4961) (55.5098, -36.3478) knots 0 0 0 1 2 2 2 projected
  spline S129 degree 2 poles (55.5098, -36.3478) (55.2428, -36.1995) (54.7188, -35.7694) (54.4667, -35.5322) knots 0 0 0 1 2 2 2 projected
  spline S130 degree 2 poles (54.4667, -35.5322) (54.0466, -35.1466) (53.1469, -34.2024) (52.8849, -33.9207) knots 0 0 0 1 2 2 2 projected
  line L166 (52.8849, -33.9207) -> (52.8849, -36.9163) projected
  line L167 (46.712, 24.6769) -> (42.1345, 24.6769) projected
  line L168 (42.1345, 24.6769) -> (42.1345, 25.4481) projected
  line L169 (42.1345, 25.4481) -> (42.6387, 25.4481) projected
  spline S131 degree 2 poles (42.6387, 25.4481) (42.3273, 25.804) (42.006, 26.4417) (42.006, 26.8371) knots 0 0 0 1 2 2 2 projected
  spline S132 degree 2 poles (42.006, 26.8371) (42.006, 27.1337) (42.2037, 27.6626) (42.4163, 27.8554) knots 0 0 0 1 2 2 2 projected
  spline S133 degree 2 poles (42.4163, 27.8554) (42.6288, 28.0532) (43.2764, 28.2707) (43.7411, 28.2707) knots 0 0 0 1 2 2 2 projected
  line L170 (43.7411, 28.2707) -> (46.712, 28.2707) projected
  line L171 (46.712, 28.2707) -> (46.712, 27.4995) projected
  line L172 (46.712, 27.4995) -> (44.1019, 27.4995) projected
  spline S134 degree 2 poles (44.1019, 27.4995) (43.7361, 27.4995) (43.2566, 27.4451) (43.0787, 27.3512) knots 0 0 0 1 2 2 2 projected
  spline S135 degree 2 poles (43.0787, 27.3512) (42.9007, 27.2573) (42.7376, 26.936) (42.7376, 26.6344) knots 0 0 0 1 2 2 2 projected
  spline S136 degree 2 poles (42.7376, 26.6344) (42.7376, 26.3527) (43.0589, 25.715) (43.2912, 25.4481) knots 0 0 0 1 2 2 2 projected
  line L173 (43.2912, 25.4481) -> (46.712, 25.4481) projected
  line L174 (46.712, 25.4481) -> (46.712, 24.6769) projected
  line L175 (48.5064, 19.966) -> (42.1345, 19.966) projected
  line L176 (42.1345, 19.966) -> (42.1345, 20.7371) projected
  line L177 (42.1345, 20.7371) -> (48.5064, 20.7371) projected
  line L178 (48.5064, 20.7371) -> (48.5064, 19.966) projected
  line L179 (48.2345, 3.4851) -> (42.1345, 3.4851) projected
  line L180 (42.1345, 3.4851) -> (42.1345, 4.2958) projected
  line L181 (42.1345, 4.2958) -> (47.3892, 4.2958) projected
  line L182 (47.3892, 4.2958) -> (43.8152, 5.8875) projected
  line L183 (43.8152, 5.8875) -> (43.8152, 6.3819) projected
  line L184 (43.8152, 6.3819) -> (47.3892, 7.9588) projected
  line L185 (47.3892, 7.9588) -> (42.1345, 7.9588) projected
  line L186 (42.1345, 7.9588) -> (42.1345, 8.7151) projected
  line L187 (42.1345, 8.7151) -> (48.2345, 8.7151) projected
  line L188 (48.2345, 8.7151) -> (48.2345, 7.6078) projected
  line L189 (48.2345, 7.6078) -> (44.8385, 6.0853) projected
  line L190 (44.8385, 6.0853) -> (48.2345, 4.6122) projected
  line L191 (48.2345, 4.6122) -> (48.2345, 3.4851) projected
  line L192 (46.6873, -7.3308) -> (45.8865, -7.3308) projected
  line L193 (45.8865, -7.3308) -> (45.8865, -7.2912) projected
  spline S137 degree 2 poles (45.8865, -7.2912) (45.9112, -7.2023) (45.9211, -7.0095) (45.9211, -6.876) knots 0 0 0 1 2 2 2 projected
  spline S138 degree 2 poles (45.9211, -6.876) (45.9211, -6.5646) (45.6492, -5.9516) (45.3822, -5.6748) knots 0 0 0 1 2 2 2 projected
  line L194 (45.3822, -5.6748) -> (42.1345, -5.6748) projected
  line L195 (42.1345, -5.6748) -> (42.1345, -4.9036) projected
  line L196 (42.1345, -4.9036) -> (46.712, -4.9036) projected
  line L197 (46.712, -4.9036) -> (46.712, -5.6748) projected
  line L198 (46.712, -5.6748) -> (46.0298, -5.6748) projected
  spline S139 degree 2 poles (46.0298, -5.6748) (46.4055, -6.095) (46.712, -6.7228) (46.712, -7.0194) knots 0 0 0 1 2 2 2 projected
  spline S140 degree 2 poles (46.712, -7.0194) (46.712, -7.138) (46.7021, -7.2566) (46.6873, -7.3308) knots 0 0 0 1 2 2 2 projected
  line L199 (48.2741, -8.7693) -> (47.4732, -8.7693) projected
  line L200 (47.4732, -8.7693) -> (47.4732, -7.8943) projected
  line L201 (47.4732, -7.8943) -> (48.2741, -7.8943) projected
  line L202 (48.2741, -7.8943) -> (48.2741, -8.7693) projected
  line L203 (44.8879, -20.4305) -> (44.2305, -20.4305) projected
  line L204 (44.2305, -20.4305) -> (44.2305, -19.7038) projected
  line L205 (44.2305, -19.7038) -> (42.1345, -19.7038) projected
  line L206 (42.1345, -19.7038) -> (42.1345, -18.9178) projected
  line L207 (42.1345, -18.9178) -> (44.2305, -18.9178) projected
  line L208 (44.2305, -18.9178) -> (44.2305, -16.2237) projected
  line L209 (44.2305, -16.2237) -> (45.0906, -16.2237) projected
  line L210 (45.0906, -16.2237) -> (48.2345, -18.9524) projected
  line L211 (48.2345, -18.9524) -> (48.2345, -19.7038) projected
  line L212 (48.2345, -19.7038) -> (44.8879, -19.7038) projected
  line L213 (44.8879, -19.7038) -> (44.8879, -20.4305) projected
  line L214 (44.4529, -23.174) -> (42.1345, -24.7509) projected
  line L215 (42.1345, -24.7509) -> (42.1345, -23.8067) projected
  line L216 (42.1345, -23.8067) -> (43.8548, -22.6945) projected
  line L217 (43.8548, -22.6945) -> (42.1345, -21.5526) projected
  line L218 (42.1345, -21.5526) -> (42.1345, -20.6776) projected
  line L219 (42.1345, -20.6776) -> (44.4035, -22.2644) projected
  line L220 (44.4035, -22.2644) -> (46.712, -20.6925) projected
  line L221 (46.712, -20.6925) -> (46.712, -21.6366) projected
  line L222 (46.712, -21.6366) -> (45.0065, -22.7439) projected
  line L223 (45.0065, -22.7439) -> (46.712, -23.8759) projected
  line L224 (46.712, -23.8759) -> (46.712, -24.7509) projected
  line L225 (46.712, -24.7509) -> (44.4529, -23.174) projected
  line L226 (-28.4263, -62.0535) -> (-29.0838, -62.0535) projected
  line L227 (-29.0838, -62.0535) -> (-29.0838, -61.3269) projected
  line L228 (-29.0838, -61.3269) -> (-31.1797, -61.3269) projected
  line L229 (-31.1797, -61.3269) -> (-31.1797, -60.5409) projected
  line L230 (-31.1797, -60.5409) -> (-29.0838, -60.5409) projected
  line L231 (-29.0838, -60.5409) -> (-29.0838, -57.8468) projected
  line L232 (-29.0838, -57.8468) -> (-28.2237, -57.8468) projected
  line L233 (-28.2237, -57.8468) -> (-25.0797, -60.5755) projected
  line L234 (-25.0797, -60.5755) -> (-25.0797, -61.3269) projected
  line L235 (-25.0797, -61.3269) -> (-28.4263, -61.3269) projected
  line L236 (-28.4263, -61.3269) -> (-28.4263, -62.0535) projected
  line L237 (-13.3524, -61.8154) -> (-14.0593, -61.8154) projected
  line L238 (-14.0593, -61.8154) -> (-14.0593, -58.0535) projected
  line L239 (-14.0593, -58.0535) -> (-13.1942, -58.0535) projected
  spline S141 degree 2 poles (-13.1942, -58.0535) (-12.8136, -58.4589) (-12.1067, -59.1806) (-11.7261, -59.5266) knots 0 0 0 1 2 2 2 projected
  spline S142 degree 2 poles (-11.7261, -59.5266) (-10.9599, -60.2236) (-10.0404, -60.7328) (-9.551, -60.7328) knots 0 0 0 1 2 2 2 projected
  spline S143 degree 2 poles (-9.551, -60.7328) (-9.294, -60.7328) (-8.9084, -60.5746) (-8.7848, -60.4312) knots 0 0 0 1 2 2 2 projected
  spline S144 degree 2 poles (-8.7848, -60.4312) (-8.6612, -60.2879) (-8.5377, -59.9122) (-8.5377, -59.6848) knots 0 0 0 1 2 2 2 projected
  spline S145 degree 2 poles (-8.5377, -59.6848) (-8.5377, -59.4673) (-8.6464, -59.0224) (-8.7305, -58.8197) knots 0 0 0 1 2 2 2 projected
  spline S146 degree 2 poles (-8.7305, -58.8197) (-8.7997, -58.6467) (-8.9974, -58.3254) (-9.0666, -58.2265) knots 0 0 0 1 2 2 2 projected
  line L240 (-9.0666, -58.2265) -> (-9.0666, -58.1821) projected
  line L241 (-9.0666, -58.1821) -> (-8.1966, -58.1821) projected
  spline S147 degree 2 poles (-8.1966, -58.1821) (-8.073, -58.4342) (-7.8308, -59.3388) (-7.8308, -59.7441) knots 0 0 0 1 2 2 2 projected
  spline S148 degree 2 poles (-7.8308, -59.7441) (-7.8308, -60.5993) (-8.7354, -61.5633) (-9.5065, -61.5633) knots 0 0 0 1 2 2 2 projected
  spline S149 degree 2 poles (-9.5065, -61.5633) (-9.8674, -61.5633) (-10.4705, -61.3952) (-10.7275, -61.2469) knots 0 0 0 1 2 2 2 projected
  spline S150 degree 2 poles (-10.7275, -61.2469) (-10.9945, -61.0986) (-11.5185, -60.6685) (-11.7706, -60.4312) knots 0 0 0 1 2 2 2 projected
  spline S151 degree 2 poles (-11.7706, -60.4312) (-12.1907, -60.0457) (-13.0904, -59.1015) (-13.3524, -58.8197) knots 0 0 0 1 2 2 2 projected
  line L242 (-13.3524, -58.8197) -> (-13.3524, -61.8154) projected
  spline S152 degree 2 poles (-6.7418, 59.8004) (-6.638, 59.9537) (-6.554, 60.3294) (-6.554, 60.5419) knots 0 0 0 1 2 2 2 projected
  spline S153 degree 2 poles (-6.554, 60.5419) (-6.554, 60.7644) (-6.6627, 61.2043) (-6.7467, 61.4169) knots 0 0 0 1 2 2 2 projected
  spline S154 degree 2 poles (-6.7467, 61.4169) (-6.8308, 61.6146) (-7.0087, 61.9063) (-7.0878, 62.02) knots 0 0 0 1 2 2 2 projected
  line L243 (-7.0878, 62.02) -> (-7.0878, 62.0694) projected
  line L244 (-7.0878, 62.0694) -> (-6.2228, 62.0694) projected
  spline S155 degree 2 poles (-6.2228, 62.0694) (-6.0794, 61.8025) (-5.8471, 60.888) (-5.8471, 60.4777) knots 0 0 0 1 2 2 2 projected
  spline S156 degree 2 poles (-5.8471, 60.4777) (-5.8471, 60.0624) (-6.0151, 59.4445) (-6.1931, 59.1924) knots 0 0 0 1 2 2 2 projected
  spline S157 degree 2 poles (-6.1931, 59.1924) (-6.3859, 58.9255) (-6.9445, 58.6487) (-7.3202, 58.6487) knots 0 0 0 1 2 2 2 projected
  spline S158 degree 2 poles (-7.3202, 58.6487) (-7.8244, 58.6487) (-8.5856, 59.3111) (-8.6845, 59.7757) knots 0 0 0 1 2 2 2 projected
  line L245 (-8.6845, 59.7757) -> (-8.7438, 59.7757) projected
  spline S159 degree 2 poles (-8.7438, 59.7757) (-8.7834, 59.5829) (-8.9613, 59.143) (-9.1393, 58.9551) knots 0 0 0 1 2 2 2 projected
  spline S160 degree 2 poles (-9.1393, 58.9551) (-9.3123, 58.7673) (-9.866, 58.53) (-10.2664, 58.53) knots 0 0 0 1 2 2 2 projected
  spline S161 degree 2 poles (-10.2664, 58.53) (-10.6767, 58.53) (-11.3737, 58.8118) (-11.6406, 59.0688) knots 0 0 0 1 2 2 2 projected
  spline S162 degree 2 poles (-11.6406, 59.0688) (-11.9174, 59.3358) (-12.2041, 60.0921) (-12.2041, 60.5716) knots 0 0 0 1 2 2 2 projected
  spline S163 degree 2 poles (-12.2041, 60.5716) (-12.2041, 61.0313) (-11.9817, 61.931) (-11.8284, 62.2375) knots 0 0 0 1 2 2 2 projected
  line L246 (-11.8284, 62.2375) -> (-10.9634, 62.2375) projected
  line L247 (-10.9634, 62.2375) -> (-10.9634, 62.1782) projected
  spline S164 degree 2 poles (-10.9634, 62.1782) (-11.1512, 61.9211) (-11.4972, 61.0511) (-11.4972, 60.621) knots 0 0 0 1 2 2 2 projected
  spline S165 degree 2 poles (-11.4972, 60.621) (-11.4972, 60.3689) (-11.339, 59.8647) (-11.1561, 59.6966) knots 0 0 0 1 2 2 2 projected
  spline S166 degree 2 poles (-11.1561, 59.6966) (-10.9732, 59.5335) (-10.5382, 59.3605) (-10.207, 59.3605) knots 0 0 0 1 2 2 2 projected
  spline S167 degree 2 poles (-10.207, 59.3605) (-9.8758, 59.3605) (-9.4458, 59.5533) (-9.3222, 59.7263) knots 0 0 0 1 2 2 2 projected
  spline S168 degree 2 poles (-9.3222, 59.7263) (-9.1986, 59.8993) (-9.1047, 60.3689) (-9.1047, 60.6457) knots 0 0 0 1 2 2 2 projected
  line L248 (-9.1047, 60.6457) -> (-9.1047, 60.9918) projected
  line L249 (-9.1047, 60.9918) -> (-8.4275, 60.9918) projected
  line L250 (-8.4275, 60.9918) -> (-8.4275, 60.7199) projected
  spline S169 degree 2 poles (-8.4275, 60.7199) (-8.4275, 60.1712) (-7.9035, 59.4791) (-7.4042, 59.4791) knots 0 0 0 1 2 2 2 projected
  spline S170 degree 2 poles (-7.4042, 59.4791) (-7.1719, 59.4791) (-6.8407, 59.6571) (-6.7418, 59.8004) knots 0 0 0 1 2 2 2 projected
  line L251 (25.6799, 59.1531) -> (25.057, 59.1531) projected
  line L252 (25.057, 59.1531) -> (25.057, 62.129) projected
  line L253 (25.057, 62.129) -> (25.6799, 62.129) projected
  line L254 (25.6799, 62.129) -> (25.6799, 61.0217) projected
  line L255 (25.6799, 61.0217) -> (29.768, 61.0217) projected
  line L256 (29.768, 61.0217) -> (29.768, 62.129) projected
  line L257 (29.768, 62.129) -> (30.3266, 62.129) projected
  spline S171 degree 2 poles (30.3266, 62.129) (30.3266, 61.5012) (30.6825, 60.908) (31.1768, 60.8684) knots 0 0 0 1 2 2 2 projected
  line L258 (31.1768, 60.8684) -> (31.1768, 60.2357) projected
  line L259 (31.1768, 60.2357) -> (25.6799, 60.2357) projected
  line L260 (25.6799, 60.2357) -> (25.6799, 59.1531) projected
  line L261 (7.2806, 58.5635) -> (6.5737, 58.5635) projected
  line L262 (6.5737, 58.5635) -> (6.5737, 62.3253) projected
  line L263 (6.5737, 62.3253) -> (7.4388, 62.3253) projected
  spline S172 degree 2 poles (7.4388, 62.3253) (7.8194, 61.9199) (8.5263, 61.1982) (8.9069, 60.8522) knots 0 0 0 1 2 2 2 projected
  spline S173 degree 2 poles (8.9069, 60.8522) (9.6731, 60.1552) (10.5926, 59.646) (11.0819, 59.646) knots 0 0 0 1 2 2 2 projected
  spline S174 degree 2 poles (11.0819, 59.646) (11.339, 59.646) (11.7246, 59.8042) (11.8482, 59.9476) knots 0 0 0 1 2 2 2 projected
  spline S175 degree 2 poles (11.8482, 59.9476) (11.9717, 60.0909) (12.0953, 60.4666) (12.0953, 60.694) knots 0 0 0 1 2 2 2 projected
  spline S176 degree 2 poles (12.0953, 60.694) (12.0953, 60.9115) (11.9866, 61.3564) (11.9025, 61.5591) knots 0 0 0 1 2 2 2 projected
  spline S177 degree 2 poles (11.9025, 61.5591) (11.8333, 61.7321) (11.6356, 62.0534) (11.5664, 62.1523) knots 0 0 0 1 2 2 2 projected
  line L264 (11.5664, 62.1523) -> (11.5664, 62.1968) projected
  line L265 (11.5664, 62.1968) -> (12.4364, 62.1968) projected
  spline S178 degree 2 poles (12.4364, 62.1968) (12.56, 61.9447) (12.8022, 61.04) (12.8022, 60.6347) knots 0 0 0 1 2 2 2 projected
  spline S179 degree 2 poles (12.8022, 60.6347) (12.8022, 59.7795) (11.8976, 58.8156) (11.1264, 58.8156) knots 0 0 0 1 2 2 2 projected
  spline S180 degree 2 poles (11.1264, 58.8156) (10.7656, 58.8156) (10.1625, 58.9836) (9.9054, 59.1319) knots 0 0 0 1 2 2 2 projected
  spline S181 degree 2 poles (9.9054, 59.1319) (9.6385, 59.2802) (9.1145, 59.7103) (8.8624, 59.9476) knots 0 0 0 1 2 2 2 projected
  spline S182 degree 2 poles (8.8624, 59.9476) (8.4422, 60.3331) (7.5426, 61.2773) (7.2806, 61.5591) knots 0 0 0 1 2 2 2 projected
  line L266 (7.2806, 61.5591) -> (7.2806, 58.5635) projected
  line L267 (-28.0763, 58.3253) -> (-28.7338, 58.3253) projected
  line L268 (-28.7338, 58.3253) -> (-28.7338, 59.0519) projected
  line L269 (-28.7338, 59.0519) -> (-30.8297, 59.0519) projected
  line L270 (-30.8297, 59.0519) -> (-30.8297, 59.8379) projected
  line L271 (-30.8297, 59.8379) -> (-28.7338, 59.8379) projected
  line L272 (-28.7338, 59.8379) -> (-28.7338, 62.532) projected
  line L273 (-28.7338, 62.532) -> (-27.8736, 62.532) projected
  line L274 (-27.8736, 62.532) -> (-24.7297, 59.8033) projected
  line L275 (-24.7297, 59.8033) -> (-24.7297, 59.0519) projected
  line L276 (-24.7297, 59.0519) -> (-28.0763, 59.0519) projected
  line L277 (-28.0763, 59.0519) -> (-28.0763, 58.3253) projected
  line L278 (25.3299, -61.2257) -> (24.707, -61.2257) projected
  line L279 (24.707, -61.2257) -> (24.707, -58.2498) projected
  line L280 (24.707, -58.2498) -> (25.3299, -58.2498) projected
  line L281 (25.3299, -58.2498) -> (25.3299, -59.3571) projected
  line L282 (25.3299, -59.3571) -> (29.418, -59.3571) projected
  line L283 (29.418, -59.3571) -> (29.418, -58.2498) projected
  line L284 (29.418, -58.2498) -> (29.9765, -58.2498) projected
  spline S183 degree 2 poles (29.9765, -58.2498) (29.9765, -58.8776) (30.3325, -59.4708) (30.8268, -59.5104) knots 0 0 0 1 2 2 2 projected
  line L285 (30.8268, -59.5104) -> (30.8268, -60.1431) projected
  line L286 (30.8268, -60.1431) -> (25.3299, -60.1431) projected
  line L287 (25.3299, -60.1431) -> (25.3299, -61.2257) projected
  spline S184 degree 2 poles (9.6836, -59.9684) (9.7874, -59.8151) (9.8714, -59.4394) (9.8714, -59.2269) knots 0 0 0 1 2 2 2 projected
  spline S185 degree 2 poles (9.8714, -59.2269) (9.8714, -59.0044) (9.7627, -58.5645) (9.6786, -58.3519) knots 0 0 0 1 2 2 2 projected
  spline S186 degree 2 poles (9.6786, -58.3519) (9.5946, -58.1542) (9.4166, -57.8625) (9.3375, -57.7488) knots 0 0 0 1 2 2 2 projected
  line L288 (9.3375, -57.7488) -> (9.3375, -57.6994) projected
  line L289 (9.3375, -57.6994) -> (10.2026, -57.6994) projected
  spline S187 degree 2 poles (10.2026, -57.6994) (10.346, -57.9663) (10.5783, -58.8808) (10.5783, -59.2911) knots 0 0 0 1 2 2 2 projected
  spline S188 degree 2 poles (10.5783, -59.2911) (10.5783, -59.7064) (10.4102, -60.3243) (10.2323, -60.5764) knots 0 0 0 1 2 2 2 projected
  spline S189 degree 2 poles (10.2323, -60.5764) (10.0395, -60.8433) (9.4809, -61.1201) (9.1052, -61.1201) knots 0 0 0 1 2 2 2 projected
  spline S190 degree 2 poles (9.1052, -61.1201) (8.601, -61.1201) (7.8397, -60.4577) (7.7409, -59.9931) knots 0 0 0 1 2 2 2 projected
  line L290 (7.7409, -59.9931) -> (7.6815, -59.9931) projected
  spline S191 degree 2 poles (7.6815, -59.9931) (7.642, -60.1859) (7.464, -60.6258) (7.2861, -60.8137) knots 0 0 0 1 2 2 2 projected
  spline S192 degree 2 poles (7.2861, -60.8137) (7.1131, -61.0015) (6.5594, -61.2388) (6.159, -61.2388) knots 0 0 0 1 2 2 2 projected
  spline S193 degree 2 poles (6.159, -61.2388) (5.7487, -61.2388) (5.0517, -60.957) (4.7848, -60.7) knots 0 0 0 1 2 2 2 projected
  spline S194 degree 2 poles (4.7848, -60.7) (4.508, -60.433) (4.2212, -59.6767) (4.2212, -59.1972) knots 0 0 0 1 2 2 2 projected
  spline S195 degree 2 poles (4.2212, -59.1972) (4.2212, -58.7375) (4.4437, -57.8378) (4.5969, -57.5313) knots 0 0 0 1 2 2 2 projected
  line L291 (4.5969, -57.5313) -> (5.462, -57.5313) projected
  line L292 (5.462, -57.5313) -> (5.462, -57.5906) projected
  spline S196 degree 2 poles (5.462, -57.5906) (5.2742, -57.8477) (4.9281, -58.7177) (4.9281, -59.1478) knots 0 0 0 1 2 2 2 projected
  spline S197 degree 2 poles (4.9281, -59.1478) (4.9281, -59.3999) (5.0863, -59.9041) (5.2692, -60.0722) knots 0 0 0 1 2 2 2 projected
  spline S198 degree 2 poles (5.2692, -60.0722) (5.4521, -60.2353) (5.8871, -60.4083) (6.2183, -60.4083) knots 0 0 0 1 2 2 2 projected
  spline S199 degree 2 poles (6.2183, -60.4083) (6.5495, -60.4083) (6.9796, -60.2155) (7.1032, -60.0425) knots 0 0 0 1 2 2 2 projected
  spline S200 degree 2 poles (7.1032, -60.0425) (7.2268, -59.8695) (7.3207, -59.3999) (7.3207, -59.1231) knots 0 0 0 1 2 2 2 projected
  line L293 (7.3207, -59.1231) -> (7.3207, -58.777) projected
  line L294 (7.3207, -58.777) -> (7.9979, -58.777) projected
  line L295 (7.9979, -58.777) -> (7.9979, -59.0489) projected
  spline S201 degree 2 poles (7.9979, -59.0489) (7.9979, -59.5976) (8.5219, -60.2897) (9.0212, -60.2897) knots 0 0 0 1 2 2 2 projected
  spline S202 degree 2 poles (9.0212, -60.2897) (9.2535, -60.2897) (9.5847, -60.1117) (9.6836, -59.9684) knots 0 0 0 1 2 2 2 projected
  arc A0 (61, 64.5) -> (60, 65.5) centre (60, 64.5) ccw projected
  line L296 (60, 65.5) -> (-60, 65.5) projected
  arc A1 (-60, 65.5) -> (-61, 64.5) centre (-60, 64.5) ccw projected
  line L297 (-61, 64.5) -> (-61, -64.5) projected
  arc A2 (-61, -64.5) -> (-60, -65.5) centre (-60, -64.5) ccw projected
  line L298 (-60, -65.5) -> (60, -65.5) projected
  arc A3 (60, -65.5) -> (61, -64.5) centre (60, -64.5) ccw projected
  line L299 (61, -64.5) -> (61, 64.5) projected
  circle A4 centre (-52.5, 57) radius 1.5 projected
  circle A5 centre (52.5, -57) radius 1.5 projected
  circle A6 centre (-52.5, -57) radius 1.5 projected
  circle A7 centre (52.5, 57) radius 1.5 projected
  line L300 (64, 15) -> (-64, 15)
  line L301 (-64, 15) -> (-64, -15)
  line L302 (-64, -15) -> (64, -15)
  line L303 (64, -15) -> (64, 15)
  line L304 (64, 15) -> (-64, -15) construction
  line L305 (-64, 15) -> (64, -15) construction
  line L306 (30, 15) -> (-30, 15)
  line L307 (-30, 15) -> (-30, -45)
  line L308 (-30, -45) -> (30, -45)
  line L309 (30, -45) -> (30, 15)
  line L310 (30, 15) -> (-30, -45) construction
  line L311 (-30, 15) -> (30, -45) construction
  point P0 (0, 0)
  point P1 (0, -15)
  point P2 (30, -15)
  point P3 (-30, -15)
  dimension "d0" = 128
  dimension "d1" = 30
  dimension "d29" = 60
  dimension "d30" = 60
  constraints: 24 end point, 5 midpoint, 4 parallel, 2 horizontal, 2 perpendicular
  measures "d0" distance of L302.end L301.end
  measures "d1" distance of L301.end L300.end
  measures "d29" distance of L308.end L307.end
  measures "d30" distance of L307.end L306.end
extrude "Extrusion1" add sketch "Sketch1" along normal blind 4 contours L11 L12 L13 L14 L15 L16 L17 L18 L19 L20 L21 L22 | L23 L24 L25 L26 | S0 S1 L27 L28 L29 L30 L31 L32 L33 L34 L35 L36 L37 S2 S3 S4 L38 L39 | L40 S5 S6 S7 S8 S9 S10 L41 S11 S12 S13 L42 L43 S14 S15 S16 L44 L45 | L46 L47 S17 S18 L48 L49 L50 L51 L52 S19 S20 | L302 L85 L86 L87 | L87 L86 L85 L302 L309 L300 S74 S73 L134 L133 L132 L299 | L299 L300 L303 L302 | L309 L308 L307 L302 | L302 L307 L300 L309 | L302 L297 L300 L307 | L132 L133 L134 L300 | L302 L301 L300 L297 | L300 S73 S74 | L88 L89 L90 L91 L92 L93 L94 L95 L96 L97 L98 L99 | L100 L101 L102 L103 L104 L105 L106 S52 L107 L108 L109 | S86 S87 S88 S89 | L136 L137 L138 L139 | S90 S91 L140 L141 S92 S93 S94 S95 S96 S97 S98 S99 L142 L143 S100 S101 S102 S103 S104 S105 | L179 L180 L181 L182 L183 L184 L185 L186 L187 L188 L189 L190 L191 | L192 L193 S137 S138 L194 L195 L196 L197 L198 S139 S140 | L199 L200 L201 L202
sketch "Sketch2" plane through (0, 0, 0) normal (0, 0, -1) x (-1, 0, 0)
  line L0 (-61, -64.5) -> (-61, 64.5) projected
  line L1 (61, 64.5) -> (61, -64.5) projected
  line L2 (-64, 15) -> (64, 15) projected
  line L3 (64, -15) -> (-64, -15) projected
  line L4 (64, 15) -> (61, 15)
  line L5 (61, 15) -> (61, -15)
  line L6 (61, -15) -> (64, -15)
  line L7 (64, -15) -> (64, 15)
  line L8 (-64, -15) -> (-64, 15) projected
  line L9 (-64, 15) -> (-61, 15)
  line L10 (-61, 15) -> (-61, -15)
  line L11 (-61, -15) -> (-64, -15)
  line L12 (-64, -15) -> (-64, 15)
  point P0 (0, 0)
  point P1 (61, 15)
  point P2 (-61, -15)
  point P3 (-61, 15)
  constraints: 16 end point, 4 parallel, 4 point on line, 2 horizontal, 2 perpendicular
extrude "Extrusion2" add sketch "Sketch2" along normal blind 21 contours L3 L8 L2 L0 | L1 L2 L7 L3
sketch "Sketch3" plane through (61, -15, 0) normal (-1, 0, 0) x (0, 0, 1)
  line L0 (-18.5, -33) -> (-18.5, 63) projected
  line L1 (-21, 0) -> (-21, 30) projected
  line L2 (-21, 30) -> (-18.5, 30)
  line L3 (-18.5, 30) -> (-18.5, 0)
  line L4 (-18.5, 0) -> (-21, 0)
  line L5 (-21, 0) -> (-21, 30)
  point P0 (0, 15)
  constraints: 8 end point, 2 parallel, 1 horizontal, 1 perpendicular, 1 point on line
extrude "Extrusion3" add sketch "Sketch3" along normal blind 3
sketch "Sketch4" plane through (-61, -15, 0) normal (1, 0, 0) x (0, 0, -1)
  line L0 (18.5, 63) -> (18.5, -33) projected
  line L1 (21, 30) -> (21, 0) projected
  line L2 (21, 30) -> (18.5, 30)
  line L3 (18.5, 30) -> (18.5, 0)
  line L4 (18.5, 0) -> (21, 0)
  line L5 (21, 0) -> (21, 30)
  point P0 (0, 15)
  constraints: 8 end point, 2 parallel, 1 horizontal, 1 perpendicular, 1 point on line
extrude "Extrusion4" add sketch "Sketch4" along normal blind 3
chamfer "Chamfer1" distance 2 angle 45 2 edges at (58, 0, -21) (-58, 0, -21)
chamfer "Chamfer2" distance 1.5 angle 45 4 edges at (61, 15, -9.25) (61, -15, -9.25) (-61, -15, -9.25) (-61, 15, -9.25)
ref_plane "Work Plane1" through (0, -15, 4) normal (-1, 0, 0) x (0, 0, 1)
sketch "Sketch5" plane through (-64, -15, 4) normal (-1, 0, 0) x (0, 0, 1)
  line L0 (-25, 30) -> (0, 30) projected
  line L1 (0, 0) -> (-25, 0) projected
  line L2 (-25, 30) -> (0, 0)
  line L3 (0, 30) -> (-25, 0)
  line L4 (-16, 11.5) -> (-9, 11.5)
  line L5 (-9, 11.5) -> (-9, 18.5)
  line L6 (-9, 18.5) -> (-16, 18.5)
  line L7 (-16, 18.5) -> (-16, 11.5)
  line L8 (-16, 11.5) -> (-9, 18.5) construction
  line L9 (-9, 11.5) -> (-16, 18.5) construction
  line L10 (-25, 30) -> (-21.5, 30)
  line L11 (-21.5, 30) -> (-21.5, 26.5)
  line L12 (-21.5, 26.5) -> (-25, 26.5)
  line L13 (-25, 26.5) -> (-25, 30)
  line L14 (0, 30) -> (-3.5, 30)
  line L15 (-3.5, 30) -> (-3.5, 26.5)
  line L16 (-3.5, 26.5) -> (0, 26.5)
  line L17 (0, 26.5) -> (0, 30)
  line L18 (0, 0) -> (-3.5, 0)
  line L19 (-3.5, 0) -> (-3.5, 3.5)
  line L20 (-3.5, 3.5) -> (0, 3.5)
  line L21 (0, 3.5) -> (0, 0)
  line L22 (-25, 0) -> (-21.5, 0)
  line L23 (-21.5, 0) -> (-21.5, 3.5)
  line L24 (-21.5, 3.5) -> (-25, 3.5)
  line L25 (-25, 3.5) -> (-25, 0)
  line L26 (-21.5, 0) -> (-12.5, 11.5)
  line L27 (-12.5, 11.5) -> (-3.5, 0)
  line L28 (0, 3.5) -> (-9, 15)
  line L29 (-25, 3.5) -> (-16, 15)
  line L30 (-16, 15) -> (-25, 26.5)
  line L31 (-21.5, 30) -> (-12.5, 18.5)
  line L32 (-9, 15) -> (0, 26.5)
  line L33 (-21.5, 3.5) -> (-3.5, 3.5)
  line L34 (-3.5, 3.5) -> (-3.5, 26.5)
  line L35 (-3.5, 26.5) -> (-21.5, 26.5)
  line L36 (-21.5, 26.5) -> (-21.5, 3.5)
  line L37 (-21.5, 3.5) -> (-3.5, 26.5) construction
  line L38 (-3.5, 3.5) -> (-21.5, 26.5) construction
  line L39 (-12.5, 18.5) -> (-3.5, 30)
  point P0 (-4, 15)
  point P1 (-12.5, 15)
  point P2 (-3.5, 7.9722)
  point P3 (-3.5, 22.0278)
  point P4 (-18.7609, 3.5)
  point P5 (-6.2391, 3.5)
  point P6 (-21.5, 22.0278)
  point P7 (-21.5, 7.9722)
  point P8 (-18.7609, 26.5)
  point P9 (-6.2391, 26.5)
  dimension "d16" = 7
  dimension "d17" = 7
  dimension "d18" = 3.5
  dimension "d19" = 3.5
  dimension "d20" = 3.5
  dimension "d21" = 3.5
  dimension "d22" = 3.5
  dimension "d23" = 3.5
  dimension "d24" = 3.5
  dimension "d25" = 3.5
  constraints: 76 end point, 12 parallel, 9 midpoint, 6 horizontal, 6 perpendicular
  measures "d16" distance of L6.end L5.end
  measures "d17" distance of L5.end L4.end
  measures "d18" distance of L11.end L12.end
  measures "d19" distance of L10.end L11.end
  measures "d20" distance of L16.end L15.end
  measures "d21" distance of L15.end L14.end
  measures "d22" distance of L19.end L20.end
  measures "d23" distance of L18.end L19.end
  measures "d24" distance of L24.end L23.end
  measures "d25" distance of L23.end L22.end
extrude "Extrusion5" cut sketch "Sketch5" against normal blind 3 contours L35 L39 L31 | L30 L29 L36 | L34 L28 L32 | L27 L33 L26
fillet "Fillet1" radius 1 12 edges at (-62.5, 11.5, -2.2391) (-62.5, 11.5, -14.7609) (-62.5, 3.5, -8.5) (-62.5, 0, -5) (-62.5, 7.0278, 0.5) (-62.5, 0, -12) (-62.5, -3.5, -8.5) (-62.5, -7.0278, 0.5) (-62.5, -11.5, -2.2391) (-62.5, -11.5, -14.7609) (-62.5, 7.0278, -17.5) (-62.5, -7.0278, -17.5)
mirror "Mirror1" about plane through (0, -15, 4) normal (-1, 0, 0) of "Fillet1", "Extrusion5"
sketch "Sketch6" plane through (0, 0, 4) normal (0, 0, 1) x (1, 0, 0)
  circle A0 centre (-21.1267, -41) radius 1.5 projected
  circle A1 centre (-21.1267, -11) radius 1.5 projected
  circle A2 centre (20.8733, -11) radius 1.5 projected
  circle A3 centre (20.8733, -41) radius 1.5 projected
  point P0 (0, 0)
extrude "Extrusion6" cut sketch "Sketch6" against normal blind 4